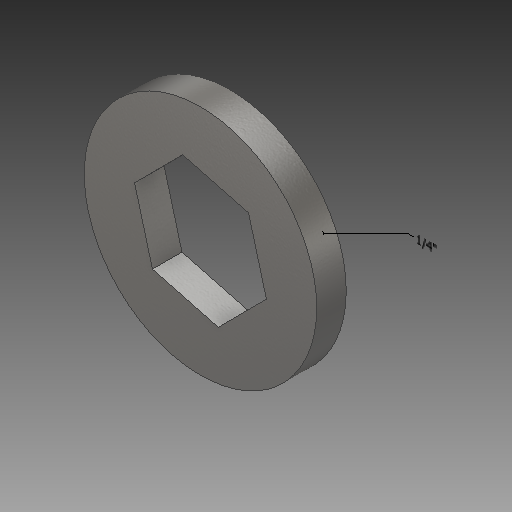
# Autodesk Inventor part: 1-4inch_KnifeSpacer_Piece1
Saved by Autodesk Inventor 2018 (Build 220112000, 112)
## iProperties
Created: 2018-01-21
Part Number: 1-4inch_KnifeSpacer_Piece1
Material: Generic
Document SubType Name: Modeling
Designer: Olivier
Density: 1 g/cm^3
Appearance: Default
Mass: 8.92029 g
Surface Area: 43.6572 cm^2
Volume: 8.92029 cm^3
Author: Olivier
Autodesk Inventor part; units mm, degrees
ref_plane "YZ Plane" through (0, 0, 0) normal (1, 0, 0) x (0, 1, 0)
ref_plane "XZ Plane" through (0, 0, 0) normal (0, 1, 0) x (-1, 0, 0)
ref_plane "XY Plane" through (0, 0, 0) normal (0, 0, 1) x (1, 0, 0)
sketch "Sketch1" plane through (0, 0, 0) normal (0, 0, 1) x (1, 0, 0)
  circle A0 centre (-75, 0) radius 25
  circle A1 centre (-75, 0) radius 25
  line L0 (-78.8445, 14.1518) -> (-64.6664, 10.4053)
  line L1 (-64.6664, 10.4053) -> (-60.8219, -3.7465)
  line L2 (-60.8219, -3.7465) -> (-71.1555, -14.1518)
  line L3 (-71.1555, -14.1518) -> (-85.3336, -10.4053)
  line L4 (-85.3336, -10.4053) -> (-89.1781, 3.7465)
  line L5 (-89.1781, 3.7465) -> (-78.8445, 14.1518)
  point P0 (0, 0)
  constraints: 12 end point, 2 centre point
extrude "Extrusion1" add sketch "Sketch1" along normal blind 6.35
body "Solid1"
